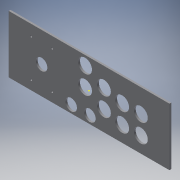
# Autodesk Inventor part: controles
Saved by Autodesk Inventor 2016 (Build 200138000, 138)
## iProperties
Created: 2017-06-07
Part Number: controles
Material: Generic
Document SubType Name: Modeling
Designer: fabio-note
Density: 1 g/cm^3
Appearance: Default
Author: fabio-note
Autodesk Inventor part; units mm, degrees
ref_plane "YZ Plane" through (0, 0, 0) normal (1, 0, 0) x (0, 1, 0)
ref_plane "XZ Plane" through (0, 0, 0) normal (0, 1, 0) x (-1, 0, 0)
ref_plane "XY Plane" through (0, 0, 0) normal (0, 0, 1) x (1, 0, 0)
sketch "Sketch1" plane through (0, 0, 0) normal (0, 1, 0) x (-1, 0, 0)
  line L0 (173, 62) -> (-173, 62)
  line L1 (-173, 62) -> (-173, -62)
  line L2 (-173, -62) -> (173, -62)
  line L3 (173, -62) -> (173, 62)
  point P0 (0, 0)
  point P1 (0, -62)
  point P2 (173, 0)
  dimension "d0" = 124
  dimension "d1" = 346
  constraints: 8 end point, 2 midpoint, 2 parallel, 1 horizontal, 1 horizontal alignment, 1 perpendicular, 1 vertical alignment
  measures "d0" distance between parallel lines of L2 L0
  measures "d1" distance between parallel lines of L1 L3
extrude "Extrusion1" add sketch "Sketch1" along normal blind 4
sketch "Esboço2" plane through (0, 0, 0) normal (0, -1, 0) x (1, 0, 0)
  circle A0 centre (111.4577, -28.224) radius 15
  circle A1 centre (71.1891, -28.224) radius 15
  circle A2 centre (71.1891, 11.776) radius 15
  circle A3 centre (111.4577, 11.776) radius 15
  circle A4 centre (31.9991, -18.8759) radius 15
  circle A5 centre (31.9991, 21.1241) radius 15
  circle A6 centre (-8.629, 1.9775) radius 15
  circle A7 centre (-8.629, 41.9775) radius 15
  circle A8 centre (1.7977, -45.4819) radius 12.5
  circle A9 centre (-38.4709, -45.4819) radius 12.5
  circle A10 centre (-102.3372, -2.2868) radius 12.5
  circle A11 centre (-79.8372, -42.1859) radius 2.25
  circle A12 centre (-124.8372, -42.1859) radius 2.25
  circle A13 centre (-79.8372, 38.8141) radius 2.1608
  circle A14 centre (-124.8372, 38.8141) radius 2.25
  point P0 (0, 0)
  dimension "d4" = 30
  dimension "d5" = 30
  dimension "d6" = 30
  dimension "d7" = 30
  dimension "d8" = 30
  dimension "d9" = 30
  dimension "d10" = 40
  dimension "d11" = 40
  dimension "d12" = 40
  dimension "d13" = 30
  dimension "d14" = 30
  dimension "d15" = 40
  dimension "d16" = 25
  dimension "d17" = 25
  dimension "d18" = 25
  dimension "d19" = 4.5
  dimension "d20" = 4.5
  dimension "d21" = 4.5
  dimension "d24" = 81
  dimension "d25" = 81
  dimension "d26" = 45
  dimension "d27" = 45
  dimension "d28" = 22.5
  constraints: 15 centre point
  measures "d4" diameter of A0
  measures "d5" diameter of A1
  measures "d6" diameter of A2
  measures "d7" diameter of A3
  measures "d8" diameter of A4
  measures "d9" diameter of A5
  measures "d10" distance of A2.centre A1.centre
  measures "d11" distance of A3.centre A0.centre
  measures "d12" distance of A5.centre A4.centre
  measures "d13" diameter of A6
  measures "d14" diameter of A7
  measures "d15" distance of A7.centre A6.centre
  measures "d16" diameter of A8
  measures "d17" diameter of A9
  measures "d18" diameter of A10
  measures "d19" diameter of A11
  measures "d20" diameter of A12
  measures "d21" diameter of A14
  measures "d24" distance of A11.centre A13.centre
  measures "d25" distance of A12.centre A14.centre
  measures "d26" distance of A11.centre A12.centre
  measures "d27" distance of A13.centre A14.centre
  measures "d28" horizontal distance of A13.centre A10.centre
extrude "Extrusão2" cut sketch "Esboço2" against normal blind 5
sketch "Esboço3" plane through (0, 0, 0) normal (0, -1, 0) x (1, 0, 0)
  point P0 (0, 0)
sketch "Esboço4" plane through (0, 4, 0) normal (0, 1, 0) x (1, 0, 0)
  line L0 (-173, -62) -> (173, -62) projected
  line L1 (-173, -62) -> (-165, -62)
  line L2 (-165, -62) -> (-165, -38)
  line L3 (-165, -38) -> (-173, -38)
  line L4 (-173, -38) -> (-173, -62)
  line L5 (-173, 62) -> (-173, -62) projected
  line L6 (-173, -12) -> (-165, -12)
  line L7 (-165, -12) -> (-165, 12)
  line L8 (-165, 12) -> (-173, 12)
  line L9 (-173, 12) -> (-173, -12)
  line L10 (-173, 38) -> (-165, 38)
  line L11 (-165, 38) -> (-165, 62)
  line L12 (-165, 62) -> (-173, 62)
  line L13 (-173, 62) -> (-173, 38)
  circle A0 centre (-165, -38) radius 1
  circle A1 centre (-165, -12) radius 1
  circle A2 centre (-165, 12) radius 1
  circle A3 centre (-165, 38) radius 1
  point P0 (0, 0)
  dimension "d29" = 8
  dimension "d30" = 24
  dimension "d31" = 24
  dimension "d32" = 26
  dimension "d33" = 24
  dimension "d34" = 26
  dimension "d37" = 2
  dimension "d38" = 2
  dimension "d39" = 2
  dimension "d40" = 2
  constraints: 24 end point, 6 parallel, 4 centre point, 4 coincident, 3 horizontal, 3 perpendicular, 2 point on line
  measures "d29" distance of L3.end L2.end
  measures "d30" distance between parallel lines of L0 L3
  measures "d31" distance between parallel lines of L6 L8
  measures "d32" distance between parallel lines of L3 L6
  measures "d33" distance between parallel lines of L12 L10
  measures "d34" distance between parallel lines of L8 L10
  measures "d37" diameter of A0
  measures "d38" diameter of A1
  measures "d39" diameter of A2
  measures "d40" diameter of A3
extrude "Extrusão3" cut sketch "Esboço4" against normal blind 10
mirror "Espelhamento1" about plane through (0, 0, 0) normal (1, 0, 0) of "Extrusão3"
body "Solid1"
